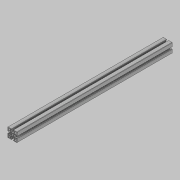
# Autodesk Inventor part: AFS-3030-200
Saved by Autodesk Inventor 2021.2 (Build 252289000, 289)
## iProperties
Created: 2016-10-06
Part Number: AFS-3030-200
Material: Generic
Document SubType Name: Modeling
Designer: gisen
Density: 1 g/cm^3
Appearance: Default
Sending System: Autodesk Inventor 2014
Preprocessor: ST-DEVELOPER v15.2
Title: C:\Users\AMS43\Documents\Inventor\AMS\misumi\フレーム_ipt\フレーム_stp\AFS-3030-6.ipt.stp
Author: AMS43
Autodesk Inventor part; units mm, degrees
ref_plane "YZ Plane" through (0, 0, 0) normal (1, 0, 0) x (0, 1, 0)
ref_plane "XZ Plane" through (0, 0, 0) normal (0, 1, 0) x (-1, 0, 0)
ref_plane "XY Plane" through (0, 0, 0) normal (0, 0, 1) x (1, 0, 0)
feature "ソリッド1" [suppressed]
sketch "スケッチ2" plane through (0, 0, 0) normal (0, 0, 1) x (1, 0, 0)
  line L0 (-12.5, 5.15) -> (-7, 5.15) projected
  line L1 (-7, 5.15) -> (-7, 3.15) projected
  line L2 (-7, 3.15) -> (-4.5, 3.15) projected
  line L3 (-4.5, 3.15) -> (-4.5, -3.15) projected
  line L4 (-4.5, -3.15) -> (-7, -3.15) projected
  line L5 (-7, -3.15) -> (-7, -5.15) projected
  line L6 (-7, -5.15) -> (-12.5, -5.15) projected
  line L7 (-12.5, -5.15) -> (-12.5, -3.15) projected
  line L8 (-12.5, -3.15) -> (-15, -3.15) projected
  line L9 (-15, -3.15) -> (-15, -14) projected
  arc A0 (-15, -14) -> (-14, -15) centre (-14, -14) ccw projected
  line L10 (-14, -15) -> (-3.15, -15) projected
  line L11 (-3.15, -15) -> (-3.15, -12.5) projected
  line L12 (-3.15, -12.5) -> (-5.15, -12.5) projected
  line L13 (-5.15, -12.5) -> (-5.15, -7) projected
  line L14 (-5.15, -7) -> (-3.15, -7) projected
  line L15 (-3.15, -7) -> (-3.15, -4.5) projected
  line L16 (-3.15, -4.5) -> (3.15, -4.5) projected
  line L17 (3.15, -4.5) -> (3.15, -7) projected
  line L18 (3.15, -7) -> (5.15, -7) projected
  line L19 (5.15, -7) -> (5.15, -12.5) projected
  line L20 (5.15, -12.5) -> (3.15, -12.5) projected
  line L21 (3.15, -12.5) -> (3.15, -15) projected
  line L22 (3.15, -15) -> (14, -15) projected
  arc A1 (14, -15) -> (15, -14) centre (14, -14) ccw projected
  line L23 (15, -14) -> (15, -3.15) projected
  line L24 (15, -3.15) -> (12.5, -3.15) projected
  line L25 (12.5, -3.15) -> (12.5, -5.15) projected
  line L26 (12.5, -5.15) -> (7, -5.15) projected
  line L27 (7, -5.15) -> (7, -3.15) projected
  line L28 (7, -3.15) -> (4.5, -3.15) projected
  line L29 (4.5, -3.15) -> (4.5, 3.15) projected
  line L30 (4.5, 3.15) -> (7, 3.15) projected
  line L31 (7, 3.15) -> (7, 5.15) projected
  line L32 (7, 5.15) -> (12.5, 5.15) projected
  line L33 (12.5, 5.15) -> (12.5, 3.15) projected
  line L34 (12.5, 3.15) -> (15, 3.15) projected
  line L35 (15, 3.15) -> (15, 14) projected
  arc A2 (15, 14) -> (14, 15) centre (14, 14) ccw projected
  line L36 (14, 15) -> (3.15, 15) projected
  line L37 (3.15, 15) -> (3.15, 12.5) projected
  line L38 (3.15, 12.5) -> (5.15, 12.5) projected
  line L39 (5.15, 12.5) -> (5.15, 7) projected
  line L40 (5.15, 7) -> (3.15, 7) projected
  line L41 (3.15, 7) -> (3.15, 4.5) projected
  line L42 (3.15, 4.5) -> (-3.15, 4.5) projected
  line L43 (-3.15, 4.5) -> (-3.15, 7) projected
  line L44 (-3.15, 7) -> (-5.15, 7) projected
  line L45 (-5.15, 7) -> (-5.15, 12.5) projected
  line L46 (-5.15, 12.5) -> (-3.15, 12.5) projected
  line L47 (-3.15, 12.5) -> (-3.15, 15) projected
  line L48 (-3.15, 15) -> (-14, 15) projected
  arc A3 (-14, 15) -> (-15, 14) centre (-14, 14) ccw projected
  line L49 (-15, 14) -> (-15, 3.15) projected
  line L50 (-15, 3.15) -> (-12.5, 3.15) projected
  line L51 (-12.5, 3.15) -> (-12.5, 5.15) projected
  circle A4 centre (10, 10) radius 3 projected
  circle A5 centre (-10, 10) radius 3 projected
  circle A6 centre (-10, -10) radius 3 projected
  circle A7 centre (10, -10) radius 3 projected
  circle A8 centre (0, 0) radius 2.5 projected
extrude "押し出し1" add sketch "スケッチ2" along normal blind 500
equation "\"d1\" = L"
equation "\"L\" = 500"
